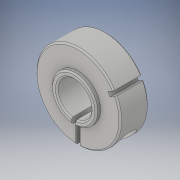
# Autodesk Inventor part: C-SCSBNAW12-16_b
Saved by Autodesk Inventor 2019 (Build 230136000, 136)
## iProperties
Created: 2023-11-30
Part Number: C-SCSBNAW12-16_b
Material: Generic
Catalog Web Link: www.cadenas.de
Description: C-SCSBNAW_base-Economy Shaft Collars - Slit
Vendor: MISUMI
Document SubType Name: Modeling
Designer: psAdmin
Manufacturer: MISUMI
Mass: 5.44517 g
Surface Area: 29.3588 cm^2
Volume: 5.44517 cm^3
Density: 1 g/cm^3
Appearance: PSOLRGB-175-175-175
Category: PARTsolutions
Company: MISUMI
Title: C-SCSBNAW12-16
Author: Cadenas PARTsolutions
Comments: Economy Shaft Collars - Slit
PSOL_IDENT_0: {$CADENAS_DATA/23d-libs/misumi/metric/03_set_collars/c_scsbnaw/c_scsbnaw_base.prj},178 {VTYP=3D},{NB=
PSOL_IDENT_1: C-SCSBNAW12-16_b},{LINA=C-SCSBNAW12-16},{NN=C-SCSBNAW_base},{DATE=12.09.2022 01:59:43},{GEOMDATE=01.
PSOL_IDENT_2: 07.2022 04:43:18},{VERSION=},{LINEID=70},{WBVAR=},{WBNUMERIC=}  {NB=C-SCSBNAW12-16_b},{LINA=C-SCSBNA
PSOL_IDENT_3: W12-16},{KT=DUMMY},{PN=C-SCSBNAW12-16},{TYPE=C-SCSBNAW},{D=12},{DSS=16},{BB=10},{B=11.5},{D1=30},{M=
PSOL_IDENT_4: M4},{THMD=4},{DD=4.5},{H=7.5},{X=10.0},{Y=5},{W=1.5},{C=0.5},{WL=2.3},{L=12}
NB: C-SCSBNAW12-16_b
NN: C-SCSBNAW_base
NT: Economy Shaft Collars - Slit Bearing Inner Mount
NBSYN: $PN._b
LINA: C-SCSBNAW12-16
CATALOG: Misumi
PN: C-SCSBNAW12-16
D: 12
DSS: 16
BB: 10
B: 11.5
D1: 30
M: M4
DD: 4.5
H: 7.5
X: 10
Y: 5
W: 1.5
C: 0.5
SUPPLIER: MISUMI
ARTICLENO: C-SCSBNAW12-16_b
BOMINFO: C-SCSBNAW12-16
CREATOR: CADENAS GmbH
Autodesk Inventor part; units mm, degrees
sketch "Sketch_1" plane through (0, 0, 0) normal (1, 0, 0) x (0, 1, 0)
  line L0 (0, -5) -> (0, 6.5)
  line L1 (7.5, 6.5) -> (6.5, 6.5)
  line L2 (6.5, 6.5) -> (6, 6)
  line L3 (6, 6) -> (6, -4.5)
  line L4 (6, -4.5) -> (6.5, -5)
  line L5 (6.5, -5) -> (14.5, -5)
  line L6 (14.5, -5) -> (15, -4.5)
  line L7 (15, -4.5) -> (15, 4.5)
  line L8 (15, 4.5) -> (14.5, 5)
  line L9 (14.5, 5) -> (8, 5)
  line L10 (8, 5) -> (8, 6)
  line L11 (8, 6) -> (7.5, 6.5)
  constraints: 24 end point
revolve "Revolution1" add sketch "Sketch_1" angle 360 about axis through (0, 0, -5) along (0, 0, -1)
sketch "Sketch_2" plane through (0, 0, 0) normal (0, 0, 1) x (1, 0, 0)
  line L0 (-0.75, -15) -> (0.75, -15)
  line L1 (0.75, -15) -> (0.75, 0)
  line L2 (0.75, 0) -> (-0.75, 0)
  line L3 (-0.75, 0) -> (-0.75, -15)
  constraints: 8 end point
extrude "Extrusion1" cut sketch "Sketch_2" along normal mid plane 23
sketch "Sketch_3" plane through (0, 0, 0) normal (0, 0, 1) x (1, 0, 0)
  line L0 (0, -10) -> (15, -10)
  line L1 (15, -10) -> (15, -13.75)
  line L2 (15, -13.75) -> (5, -13.75)
  line L3 (5, -13.75) -> (5, -12.25)
  line L4 (5, -12.25) -> (0, -12.25)
  line L5 (0, -12.25) -> (0, -10)
  line L6 (0, -10) -> (15, -10)
  constraints: 14 end point
revolve "Revolution2" cut sketch "Sketch_3" angle 360 about axis through (0, -10, 0) along (1, 0, 0)
sketch "Sketch4" plane through (-0.75, -14.4806, -5) normal (1, 0, 0) x (0, 0, -1)
  point P0 (-5, 4.4806)
hole "Hole1" at (-0.75, -10, 0) direction (-1, 0, 0) diameter 3.242 depth 15 thread size "M4x0.7" class "6H" standard "ISO Metric profile"
sketch "_____1" plane through (0, 0, 0) normal (0, 0, 1) x (1, 0, 0)
  line L0 (10.6235, 6.9995) -> (11.3735, 5.7005)
  line L1 (11.3735, 5.7005) -> (13.3654, 6.8505)
  line L2 (13.3654, 6.8505) -> (12.6154, 8.1495)
  line L3 (12.6154, 8.1495) -> (10.6235, 6.9995)
  constraints: 8 end point
extrude "Extrusion2" cut sketch "_____1" along normal mid plane 10
ref_plane "body_screw_XY" through (5, -10, 0) normal (1, 0, 0) x (0, 0, -1)
ref_plane "body_screw_YZ" through (5, -10, 0) normal (0, 0, -1) x (0, 1, 0)
ref_plane "body_screw_ZX" through (5, -10, 0) normal (0, 1, 0) x (1, 0, 0)
body "Solid1"
